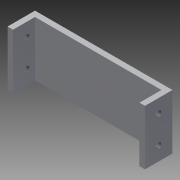
# Autodesk Inventor part: Leg_Link_Conecter
Saved by Autodesk Inventor 2013 (Build 170138000, 138)
## iProperties
Created: 2014-04-20
Part Number: Leg_Link_Conecter
Material: アルミニウム 6061
Document SubType Name: Modeling
Designer: andou
Density: 1 g/cm^3
Author: andou
Autodesk Inventor part; units mm, degrees
ref_plane "YZ Plane" through (0, 0, 0) normal (1, 0, 0) x (0, 1, 0)
ref_plane "XZ Plane" through (0, 0, 0) normal (0, 1, 0) x (-1, 0, 0)
ref_plane "XY Plane" through (0, 0, 0) normal (0, 0, 1) x (1, 0, 0)
sketch "スケッチ1" plane through (0, 0, 0) normal (0, 0, 1) x (1, 0, 0)
  line L0 (-25, 5) -> (25, 5)
  line L1 (25, 5) -> (25, -5)
  line L2 (-25, -5) -> (-25, 5)
  line L3 (-23, 3) -> (23, 3)
  line L4 (23, 3) -> (23, -5)
  line L5 (-23, -5) -> (-23, 3)
  line L6 (25, -5) -> (23, -5)
  line L7 (-23, -5) -> (-25, -5)
  point P0 (0, 0)
  dimension "d0" = 50
  dimension "d2" = 46
  dimension "d3" = 23
  dimension "d4" = 25
  dimension "d5" = 10
  dimension "d6" = 10
  dimension "d8" = 5
  dimension "d9" = 8
  constraints: 16 end point, 4 parallel, 2 horizontal, 2 perpendicular
  measures "d0" distance of L0.start L0.end
  measures "d2" distance of L3.start L3.end
  measures "d3" distance from line of point (0, 0) L5
  measures "d4" distance from line of L1 point (0, 0)
  measures "d5" distance between parallel lines of L0 L6
  measures "d6" distance between parallel lines of L0 L7
  measures "d8" distance from line of point (0, 0) L6
  measures "d9" distance between parallel lines of L3 L7
extrude "押し出し1" add sketch "スケッチ1" against normal blind 20
sketch "スケッチ2" plane through (25, -5, 0) normal (1, 0, 0) x (0, 0, -1)
  line L0 (0, 10) -> (0, 0) projected
  line L1 (0, 10) -> (20, 10) projected
  circle A0 centre (5, 5) radius 1
  circle A1 centre (15, 5) radius 1
  point P0 (0, 5)
  dimension "d14" = 5
  dimension "d15" = 5
  dimension "d16" = 5
  dimension "d17" = 10
  dimension "d18" = 2
  constraints: 2 centre point, 1 equal radius
  measures "d14" distance from line of L1 A1.centre
  measures "d15" distance from line of L1 A0.centre
  measures "d16" distance from line of L0 A0.centre
  measures "d17" distance of A1.centre A0.centre
  measures "d18" diameter of A1
hole "穴1" at (25, 0, -5) at (25, 0, -15) direction (-1, 0, 0) diameter 2 end through all
thread "ねじ3" size "M2x0.4" class "6H" standard "ANSI Metric M Profile" full length
thread "ねじ4" size "M2x0.4" class "6H" standard "ANSI Metric M Profile" full length
thread "ねじ5" size "M2x0.4" class "6H" standard "ANSI Metric M Profile" full length
thread "ねじ6" size "M2x0.4" class "6H" standard "ANSI Metric M Profile" full length
